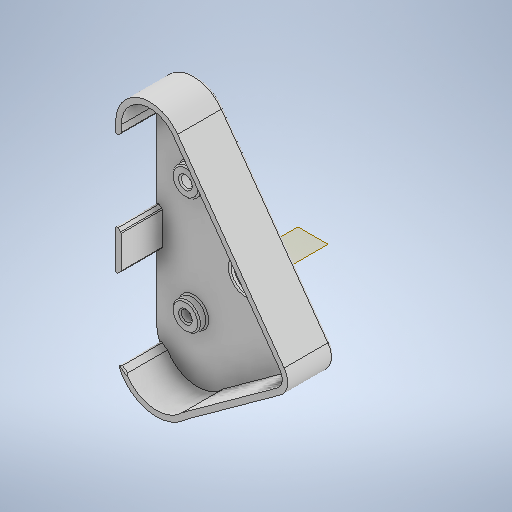
# Autodesk Inventor part: TreadWheeled
Saved by Autodesk Inventor 2025.2 (Build 292293000, 293)
## iProperties
Created: 2025-01-25
Part Number: TreadWheeled
Material: Generic
Document SubType Name: Modeling
Designer: andre
Density: 1 g/cm^3
Appearance: Default
Author: andre
## iProperties of the stored document TreadWheeled_3DPrint.ipt
Created: 2025-02-02
Part Number: TreadWheeled_3DPrint
Material: Generic
Document SubType Name: Modeling
Designer: andre
Density: 1 g/cm^3
Appearance: Default
Author: andre
Autodesk Inventor part; units mm, degrees
ref_plane "YZ Plane" through (0, 0, 0) normal (1, 0, 0) x (0, 1, 0)
ref_plane "XZ Plane" through (0, 0, 0) normal (0, 1, 0) x (-1, 0, 0)
ref_plane "XY Plane" through (0, 0, 0) normal (0, 0, 1) x (1, 0, 0)
sketch "Sketch1" plane through (0, 0, 0) normal (0, 0, 1) x (1, 0, 0)
  circle A0 centre (21.906587, -14.729638) radius 6.510732
  circle A1 centre (-22.105524, 36.567706) radius 12.5
  circle A2 centre (-19.605524, -34.582122) radius 15
  line L0 (-34.605524, 36.567706) -> (-34.605524, -34.582122)
  line L1 (27.078439, -10.774693) -> (-11.934443, 43.834006)
  line L2 (25.383273, -20.23439) -> (-8.83145, -45.018565)
  dimension "d0" = 25
  dimension "d1" = 30
  constraints: 6 end point, 6 point on circle, 3 centre point, 3 tangent, 1 vertical
  measures "d0" diameter of A1
  measures "d1" diameter of A2
extrude "Extrusion1" add sketch "Sketch1" along normal blind 17
shell "Shell1" thickness 2 removed faces 1 at (-14.044203, -2.929703, 17)
sketch "Sketch2" plane through (-32.605524, -34.582122, 2) normal (0, 0, 1) x (1, 0, 0)
  line L0 (42.323201, 12.878365) -> (42.323201, 33.588213) construction
  line L1 (19.077406, 77.206351) -> (58.077223, 22.615939) construction
  line L2 (56.871754, 16.008165) -> (22.454087, -8.923017) construction
  arc A0 (56.871754, 16.008165) -> (58.077223, 22.615939) centre (54.512111, 19.852484) ccw construction
  line L3 (13.071479, 75.291589) -> (52.429828, 20.199318) construction
  line L4 (52.429828, 20.199318) -> (18.911769, -4.080213) construction
  arc A1 (56.871754, 16.008165) -> (58.077223, 22.615939) centre (54.512111, 19.852484) ccw
  line L5 (58.077223, 22.615939) -> (19.043708, 77.25352)
  arc A2 (19.043708, 77.25352) -> (0, 71.149828) centre (10.5, 71.149828) ccw
  line L6 (0, 71.149828) -> (0, 0)
  arc A3 (0, 0) -> (22.454087, -8.923017) centre (13, 0) ccw
  line L7 (22.454087, -8.923017) -> (56.871754, 16.008165)
  line L8 (19.043708, 77.25352) -> (58.077223, 22.615939)
  line L9 (56.871754, 16.008165) -> (22.454087, -8.923017)
  circle A4 centre (42.323201, 34.346177) radius 1.75
  circle A5 centre (52.429828, 20.199318) radius 1.75
  circle A6 centre (42.323201, 12.878365) radius 1.75
  point P0 (32.605524, 34.582122)
  dimension "d5" = 6
  dimension "d7" = 3.5
  constraints: 10 end point, 5 coincident, 4 centre point, 3 point on line, 2 equal radius, 2 parallel, 2 point on circle, 1 vertical, 1 other
  measures "d5" distance between parallel lines of L1 L3
  measures "d7" diameter of A5
extrude "Extrusion2" cut sketch "Sketch2" against normal up to next contours A4 | A5 | A6
sketch "Sketch4" plane through (-32.605524, -34.582122, 2) normal (0, 0, 1) x (1, 0, 0)
  circle A0 centre (30.51356, 30.605189) radius 2.25
  circle A1 centre (30.51356, 30.605189) radius 10.204663 construction
  point P0 (32.605524, 34.582122)
  dimension "d13" = 4.5
  constraints: 2 centre point, 2 coincident
  measures "d13" diameter of A0
extrude "Extrusion3" cut sketch "Sketch4" against normal up to next
sketch "Sketch5" plane through (-32.605524, -34.582122, 2) normal (0, 0, 1) x (1, 0, 0)
  arc A0 (28.01356, 35.504169) -> (33.01356, 35.504169) centre (30.51356, 30.605189) ccw
  arc A1 (33.01356, 36.605189) -> (28.01356, 36.605189) centre (30.51356, 36.605189) ccw
  line L0 (28.01356, 36.605189) -> (28.01356, 35.504169)
  line L1 (33.01356, 35.504169) -> (33.01356, 36.605189)
  arc A2 (27.71356, 35.684559) -> (33.31356, 35.684559) centre (30.51356, 30.605189) ccw
  line L2 (27.71356, 35.684559) -> (27.71356, 36.605189)
  arc A3 (33.31356, 36.605189) -> (27.71356, 36.605189) centre (30.51356, 36.605189) ccw
  line L3 (33.31356, 36.605189) -> (33.31356, 35.684559)
  point P0 (32.605524, 34.582122)
  dimension "d39" = 0.3
  constraints: 8 end point, 8 point on circle, 4 centre point, 2 vertical, 11 other
  measures "d39" radial gap between concentric circles of A0 A2
extrude "Extrusion4" cut sketch "Sketch5" against normal up to next contours L0 A1 L1 A0 | L2 A3 L3 A2
sketch "Sketch6" plane through (-32.605524, -34.582122, 2) normal (0, 0, 1) x (1, 0, 0)
  circle A0 centre (11.539931, 52.643392) radius 5
  circle A1 centre (11.539931, 52.643392) radius 17.53054 construction
  arc A2 (27.71356, 35.684559) -> (33.31356, 35.684559) centre (30.51356, 30.605189) ccw construction
  line L0 (36.31356, 30.605189) -> (-2, 30.605189) construction
  line L1 (-2, 71.149828) -> (-2, 0) construction
  point P0 (32.605524, 34.582122)
  constraints: 2 centre point, 2 end point, 2 horizontal, 1 coincident, 1 point on circle, 1 point on line
ref_plane "Work Plane1" through (-21.29086, -23.175829, 5) normal (0, 0, -1) x (-0.6035209, 0.7973472, 0)
extrude "Extrusion5" add sketch "Sketch6" along normal up to surface (3 mm away)
sketch "Sketch7" plane through (-21.065592, 18.06127, 5) normal (0, 0, 1) x (1, 0, 0)
  circle A0 centre (0, 0) radius 5 projected
  circle A1 centre (0, 0) radius 2
  point P0 (21.065592, -18.06127)
  dimension "d22" = 4
  constraints: 1 centre point, 1 coincident
  measures "d22" diameter of A1
extrude "Extrusion6" cut sketch "Sketch7" against normal up to surface (3 mm away) contours A1
fillet "Fillet2" radius 0.5 2 edges at (-26.0656, 18.0613, 5) (-23.0656, 18.0613, 5)
sketch "Sketch10" plane through (0, 0, 17) normal (0, 0, 1) x (1, 0, 0)
  circle A0 centre (-20.109073, 17.069464) radius 17.500096 construction
  circle A1 centre (-20.108854, -25.023073) radius 17.500096
  circle A2 centre (-20.109073, 17.069464) radius 18.500096 construction
  circle A3 centre (-20.108854, -25.023073) radius 19.500096
  line L0 (-32.605524, 36.567706) -> (-32.605524, -34.582122)
  line L1 (-32.605524, 30.711027) -> (-32.605524, -39.992607)
  arc A4 (-32.605524, -34.582122) -> (-10.151436, -43.505139) centre (-19.605524, -34.582122) ccw
  circle A5 centre (-21.065592, 18.06127) radius 2
  circle A6 centre (-21.065592, 18.06127) radius 17.500096 construction
  circle A7 centre (-21.065592, 18.06127) radius 19.500096
  circle A8 centre (-20.125621, 17.055287) radius 17.500096
  point P0 (0, 0)
  point P1 (-32.605524, 3.4279)
  point P2 (-32.605524, -10.053538)
  point P3 (-30.661029, -41.421406)
  point P4 (-32.605524, 33.780167)
  point P5 (-32.605524, 2.342374)
  dimension "d33" = 1
  dimension "d34" = 2
  dimension "d43" = 35.00019
  dimension "d44" = 2
  dimension "d45" = 35.00019
  constraints: 5 centre point, 2 end point, 1 coincident, 1 collinear, 1 point on line, 12 other
  measures "d43" diameter of A6
  measures "d44" radial gap between concentric circles of A6 A7
  measures "d45" diameter of A8
extrude "Extrusion9" cut sketch "Sketch10" against normal up to surface (15 mm away) contours L0 L1 A1 | A1 L1 A3 L0 | A4 A3 L1 A1 | A1 L1 A4 | L0 A8 A7 | L0 A8 picked at (-36.467594, 27.93884) picked at (-33.403691, 20.128568)
fillet "Fillet3" radius 0.5 8 edges at (-34.0377, -38.67, 9.5) (-32.4264, -40.1403, 17) (-34.6055, -11.9808, 9.5) (-32.6055, -10.0535, 9.5) (-32.6055, 2.3424, 9.5) (-34.6055, 4.0283, 9.5) (-34.6055, 32.0942, 9.5) (-32.6055, 33.7802, 9.5)
fillet "Fillet4" radius 1 6 edges at (-34.6055, 0.9928, 0) (-25.2353, -48.4856, 0) (7.572, 16.5297, 0) (-25.9207, 48.4712, 0) (8.2759, -32.6265, 0) (28.3152, -15.8781, 0)
fillet "Fillet5" radius 0.5 10 edges at (-2.092, -9.7769, 0) (-2.092, -9.7769, 2) (-4.892, 1.5628, 0) (0.708, 1.5628, 0) (-2.092, 4.8231, 0) (0.708, 1.5628, 2) (-4.892, 1.5628, 2) (-2.092, 4.8231, 2) (-4.892, 1.1024, 1) (0.708, 1.1024, 1)
fillet "Fillet6" radius 0.5 6 edges at (7.9677, -21.7038, 2) (7.9677, -21.7038, 0) (7.9677, -0.2359, 2) (7.9677, -0.2359, 0) (18.0743, -14.3828, 0) (18.0743, -14.3828, 2)
fillet "Fillet7" radius 0.5 1 edges at (-26.0656, 18.0613, 2)
ref_plane "Work Plane5" through (3.408036, -3.226932, -22) normal (0, 1, 0) x (-1, 0, 0)
mirror "Mirror3" about plane through (3.408036, -3.226932, -22) normal (0, 1, 0) of "Fillet7", "Fillet2", "Extrusion5", "Extrusion6"
equation "\"d9\" = d7"
equation "\"d43\" = d45"
body "Solid1"
